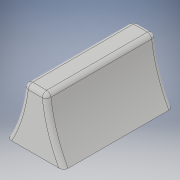
# Autodesk Inventor part: DoubleSliderCap
Saved by Autodesk Inventor 2018 (Build 220112000, 112)
## iProperties
Created: 2019-03-27
Part Number: DoubleSliderCap
Material: Generic
Document SubType Name: Modeling
Designer: matth
Density: 1 g/cm^3
Appearance: Default
Author: matth
Autodesk Inventor part; units mm, degrees
ref_plane "YZ Plane" through (0, 0, 0) normal (1, 0, 0) x (0, 1, 0)
ref_plane "XZ Plane" through (0, 0, 0) normal (0, 1, 0) x (-1, 0, 0)
ref_plane "XY Plane" through (0, 0, 0) normal (0, 0, 1) x (1, 0, 0)
sketch "Sketch1" plane through (0, 0, 0) normal (0, 0, 1) x (1, 0, 0)
  line L0 (-4.7637, 0) -> (8.2363, 0)
  line L1 (8.2363, 0) -> (8.2363, 13)
  line L2 (8.2363, 13) -> (-4.7637, 13)
  line L3 (-4.7637, 13) -> (-4.7637, 0)
  arc A0 (-4.7637, 0) -> (-0.7637, 13) centre (-33.6274, 15.9965) ccw
  arc A1 (4.2363, 13) -> (8.2363, 0) centre (37.1, 15.9965) ccw
  point P0 (0, 0)
  dimension "d0" = 13
  dimension "d1" = 13
  dimension "d2" = 4
  dimension "d3" = 4
  dimension "d4" = 33
  dimension "d5" = 33
  constraints: 8 end point, 4 point on circle, 3 perpendicular, 2 centre point, 2 point on line, 1 horizontal
  measures "d0" distance of L0.start L0.end
  measures "d1" distance of L0.end L1.end
  measures "d2" distance from line of L3 A0.end
  measures "d3" distance of L1.end A1.start
  measures "d4" radius of A0
  measures "d5" radius of A1
extrude "Extrusion1" add sketch "Sketch1" along normal blind 25 contours A0 L2 A1 L0
sketch "Sketch2" plane through (-4.7637, 0, 0) normal (0, -1, 0) x (1, 0, 0)
  line L0 (3.9, 20.185) -> (9.1, 20.185)
  line L1 (9.1, 20.185) -> (9.1, 18.785)
  line L2 (9.1, 18.785) -> (3.9, 18.785)
  line L3 (3.9, 18.785) -> (3.9, 20.185)
  line L4 (3.9, 6.215) -> (9.1, 6.215)
  line L5 (9.1, 6.215) -> (9.1, 4.815)
  line L6 (9.1, 4.815) -> (3.9, 4.815)
  line L7 (3.9, 4.815) -> (3.9, 6.215)
  line L8 (0, 0) -> (0, 25) projected
  line L9 (0, 25) -> (13, 25) projected
  point P0 (4.7637, 0)
  dimension "d8" = 5.2
  dimension "d9" = 3.9
  dimension "d10" = 1.4
  dimension "d11" = 1.4
  dimension "d12" = 15.37
  dimension "d13" = 4.815
  dimension "d23" = 13
  constraints: 16 end point, 4 parallel, 2 horizontal, 2 perpendicular, 2 point on line
  measures "d8" distance between parallel lines of L1 L3
  measures "d9" distance between parallel lines of L8 L3
  measures "d10" distance between parallel lines of L0 L2
  measures "d11" distance of L6.end L4.start
  measures "d12" distance between parallel lines of L6 L0
  measures "d13" distance between parallel lines of L9 L0
  measures "d23" distance of L8.end L9.end
extrude "Extrusion2" cut sketch "Sketch2" against normal blind 2
fillet "Fillet1" radius 1 8 edges at (4.2363, 13, 12.5) (1.7363, 13, 25) (-0.7637, 13, 12.5) (1.7363, 13, 0) (5.5593, 6.2917, 25) (-2.0867, 6.2917, 25) (5.5593, 6.2917, 0) (-2.0867, 6.2917, 0)
sketch "Sketch4" plane through (-4.7637, 2, 0) normal (0, -1, 0) x (1, 0, 0)
  point P0 (4.7637, 0)
sketch "Sketch5" plane through (-4.7637, 2, 0) normal (0, -1, 0) x (1, 0, 0)
  line L0 (3.9, 18.785) -> (9.1, 18.785) projected
  line L1 (8.6, 20.185) -> (4.4, 20.185)
  line L2 (4.4, 20.185) -> (4.4, 18.785)
  line L3 (4.4, 18.785) -> (8.6, 18.785)
  line L4 (8.6, 18.785) -> (8.6, 20.185)
  line L5 (3.9, 18.785) -> (3.9, 20.185) projected
  line L6 (9.1, 20.185) -> (9.1, 18.785) projected
  line L7 (9.1, 6.215) -> (3.9, 6.215) projected
  line L8 (4.4, 6.215) -> (8.6, 6.215)
  line L9 (8.6, 6.215) -> (8.6, 4.7558)
  line L10 (8.6, 4.7558) -> (4.4, 4.7558)
  line L11 (4.4, 4.7558) -> (4.4, 6.215)
  point P0 (4.7637, 0)
  dimension "d24" = 1.4
  dimension "d25" = 0.5
  dimension "d26" = 0.5
  constraints: 16 end point, 4 parallel, 2 horizontal, 2 perpendicular, 2 point on line
  measures "d24" distance of L1.end L2.end
  measures "d25" distance between parallel lines of L5 L2
  measures "d26" distance between parallel lines of L6 L4
extrude "Extrusion4" cut sketch "Sketch5" against normal blind 10
body "Solid1"
